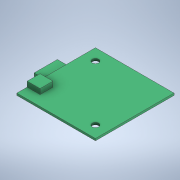
# Autodesk Inventor part: PCB
Saved by Autodesk Inventor 2022 (Build 260153000, 153)
## iProperties
Created: 2021-08-09
Part Number: PCB
Material: Ogólny
Document SubType Name: Modeling
Designer: Krystyna
Density: 3.37119 g/cm^3
Appearance: Domyślna
Mass: 25 g
Surface Area: 84.8383 cm^2
Volume: 7.41577 cm^3
Author: Krystyna
Autodesk Inventor part; units mm, degrees
ref_plane "YZ Plane" through (0, 0, 0) normal (1, 0, 0) x (0, 1, 0)
ref_plane "XZ Plane" through (0, 0, 0) normal (0, 1, 0) x (-1, 0, 0)
ref_plane "XY Plane" through (0, 0, 0) normal (0, 0, 1) x (1, 0, 0)
sketch "Szkic1" plane through (0, 0, 0) normal (0, 1, 0) x (-1, 0, 0)
  line L0 (30.5, 30.5) -> (-30.5, 30.5)
  line L1 (-30.5, 30.5) -> (-30.5, -30.5)
  line L2 (-30.5, -30.5) -> (30.5, -30.5)
  line L3 (30.5, -30.5) -> (30.5, 30.5)
  point P0 (0, 0)
  point P1 (30.5, 0)
  point P2 (0, -30.5)
  dimension "d0" = 61
  dimension "d1" = 61
  constraints: 8 end point, 2 midpoint, 2 parallel, 1 horizontal, 1 horizontal alignment, 1 perpendicular, 1 vertical alignment
  measures "d0" distance of L2.end L0.start
  measures "d1" distance of L1.end L2.end
extrude "Wyciągnięcie proste1" add sketch "Szkic1" along normal blind 1.6
sketch "Szkic2" plane through (0, 1.6, 0) normal (0, 1, 0) x (1, 0, 0)
  circle A0 centre (21.5, -21.5) radius 2.5
  circle A1 centre (-21.5, 21.5) radius 2.5
  line L0 (-30.5, -30.5) -> (30.5, -30.5) projected
  line L1 (-30.5, 30.5) -> (-30.5, -30.5) projected
  line L2 (30.5, 30.5) -> (-30.5, 30.5) projected
  line L3 (30.5, -30.5) -> (30.5, 30.5) projected
  point P0 (0, 0)
  dimension "d4" = 5
  dimension "d5" = 5
  dimension "d6" = 9
  dimension "d8" = 9
  dimension "d12" = 9
  dimension "d13" = 9
  constraints: 2 centre point
  measures "d4" diameter of A1
  measures "d5" diameter of A0
  measures "d6" distance from line of L0 A0.centre
  measures "d8" distance from line of L2 A1.centre
  measures "d12" distance from line of L3 A0.centre
  measures "d13" distance from line of L1 A1.centre
extrude "Wyciągnięcie proste2" cut sketch "Szkic2" against normal up to surface (1.6 mm away) contours A0 | A1
sketch "Szkic3" plane through (0, 0, 0) normal (0, -1, 0) x (1, 0, 0)
  line L0 (-13.9641, -9.4) -> (-38.9641, -9.4)
  line L1 (-38.9641, -9.4) -> (-38.9641, 8.6)
  line L2 (-38.9641, 8.6) -> (-13.9641, 8.6)
  line L3 (-13.9641, 8.6) -> (-13.9641, -9.4)
  line L4 (-30.5, 30.5) -> (30.5, 30.5) projected
  line L5 (-30.5, -30.5) -> (-30.5, 30.5) projected
  point P0 (0, 0)
  dimension "d14" = 18
  dimension "d15" = 25
  dimension "d16" = 21.9
  dimension "d17" = 8.4641
  constraints: 8 end point, 2 parallel, 1 horizontal, 1 perpendicular
  measures "d14" distance of L0.end L1.end
  measures "d15" distance of L0.start L0.end
  measures "d16" distance between parallel lines of L4 L2
  measures "d17" distance from line of L5 L1.end
extrude "Wyciągnięcie proste3" add sketch "Szkic3" along normal blind 2.5
sketch "Szkic4" plane through (0, 1.6, 0) normal (0, 1, 0) x (1, 0, 0)
  line L0 (-30.5, -12.5) -> (-20.5, -12.5)
  line L1 (-20.5, -12.5) -> (-20.5, -22.5)
  line L2 (-20.5, -22.5) -> (-30.5, -22.5)
  line L3 (-30.5, -22.5) -> (-30.5, -12.5)
  line L4 (-30.5, -30.5) -> (30.5, -30.5) projected
  line L5 (-30.5, 30.5) -> (-30.5, -30.5) projected
  point P0 (0, 0)
  dimension "d20" = 10
  dimension "d21" = 10
  dimension "d22" = 8
  constraints: 8 end point, 2 parallel, 1 collinear, 1 horizontal, 1 perpendicular
  measures "d20" distance of L0.end L1.end
  measures "d21" distance of L0.start L0.end
  measures "d22" distance between parallel lines of L4 L2
extrude "Wyciągnięcie proste4" add sketch "Szkic4" along normal blind 4
